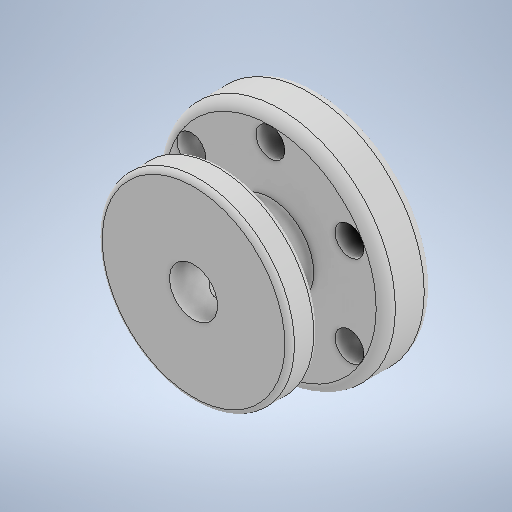
# Autodesk Inventor part: Steering Gear Plate 2
Saved by Autodesk Inventor 2025.2 (Build 292293000, 293)
## iProperties
Created: 2025-03-03
Part Number: Steering Gear Plate 2
Material: Generic
Document SubType Name: Modeling
Designer: eason
Density: 1 g/cm^3
Appearance: Default
Author: eason
Autodesk Inventor part; units mm, degrees
ref_plane "YZ Plane" through (0, 0, 0) normal (1, 0, 0) x (0, 1, 0)
sketch "Sketch1" plane through (0, 0, 0) normal (0, 0, 1) x (1, 0, 0)
  circle A0 centre (0, 0) radius 8
  circle A1 centre (0, 0) radius 11
  circle A2 centre (0, 9.5) radius 1.5
  line L0 (0, -15.4) -> (0, 15.4) projected
  circle A3 centre (-8.2272, 4.75) radius 1.5
  circle A4 centre (-8.2272, -4.75) radius 1.5
  circle A5 centre (0, -9.5) radius 1.5
  circle A6 centre (8.2272, -4.75) radius 1.5
  circle A7 centre (8.2272, 4.75) radius 1.5
  point P0 (-9.5263, 5.5)
  point P1 (-9.5263, -5.5)
  point P2 (9.5263, -5.5)
  point P3 (9.5263, 5.5)
  point P4 (0, 11)
  dimension "d0" = 16
  dimension "d1" = 22
  dimension "d4" = 360
  constraints: 8 centre point, 2 coincident, 2 tangent, 1 point on line, 13 other
  measures "d0" diameter of A0
  measures "d1" diameter of A1
extrude "Extrusion1" add sketch "Sketch1" along normal blind 5 contours A0 L0 | A0 A7 A1 A6 | A0 A2 A1 A7 | A6 A1 A5 A0 | L0 A0 | A0 A3 A1 A2 | A5 A1 A4 A0 | A5 L0 | L0 A5 | A0 A4 A1 A3
sketch "Sketch2" plane through (0, 0, 5) normal (0, 0, 1) x (1, 0, 0)
  circle A0 centre (0, 0) radius 10
  circle A1 centre (0, 0) radius 2.5
  dimension "d10" = 20
  dimension "d31" = 5
  constraints: 2 centre point, 2 coincident
  measures "d10" diameter of A0
  measures "d31" diameter of A1
extrude "Extrusion3" add sketch "Sketch2" along normal blind 8
extrude "Extrusion4" cut sketch "Sketch2" against normal through all contours A1
sketch "Sketch4" plane through (0, 0, 13) normal (0, 0, 1) x (1, 0, 0)
  line L0 (0, 0) -> (-3.4808, -9.3746) construction
  line L1 (0, -15.4) -> (0, 15.4) projected
  circle A0 centre (0, 0) radius 10 projected
  dimension "d16" = 20.37
  constraints: 2 end point, 2 other
  measures "d16" angle of L1 L0
ref_plane "Work Plane1" through (-3.4808, -9.3746, 13) normal (-0.3480812, -0.9374644, 0) x (0.9374644, -0.3480812, 0)
sketch "Sketch5" plane through (-3.4808, -9.3746, 13) normal (-0.3480812, -0.9374644, 0) x (0.9374644, -0.3480812, 0)
  circle A0 centre (0, -5) radius 1.5
  line L0 (10, 0) -> (-10, 0) projected
  line L1 (0, -15.6) -> (0, 2.6) projected
  line L2 (7.4257, -8) -> (10, -8) projected
  point P0 (0, -13)
  dimension "d17" = 3
  dimension "d33" = 3
  constraints: 1 centre point, 1 point on line
  measures "d17" diameter of A0
  measures "d33" distance from line of L2 A0.centre
extrude "Extrusion5" cut sketch "Sketch5" against normal up to surface
ref_plane "Work Plane2" through (0, 0, 9) normal (0, 0, 1) x (1, 0, 0)
sketch "Sketch6" plane through (0, 0, 9) normal (0, 0, 1) x (1, 0, 0)
  circle A0 centre (0, 0) radius 2.5 projected
  circle A1 centre (0, 0) radius 4.5
  circle A2 centre (0, 0) radius 10 projected
  dimension "d32" = 2
  constraints: 1 centre point, 1 coincident
  measures "d32" radial gap between concentric circles of A1 A0
extrude "Extrusion6" cut sketch "Sketch6" along normal blind 1 and the other way blind 4 contours A2
fillet "Fillet1" radius 0.5 6 edges at (-10, 0, 10) (-10, 0, 13) (-0.1708, -4.4968, 8.5251) (-1.5663, -4.2186, 9.5) (-2.1556, -3.9501, 6.6461) (-2.1024, -1.3528, 7.9953)
sketch "Sketch7" plane through (0, 0, 0) normal (0, 0, -1) x (-1, 0, 0)
  circle A0 centre (0, 0) radius 12
  arc A1 (9.5263, 5.5) -> (0, 11) centre (0, 0) ccw projected
  arc A2 (9.5263, -5.5) -> (9.5263, 5.5) centre (0, 0) ccw projected
  arc A3 (-9.5263, -5.5) -> (9.5263, -5.5) centre (0, 0) ccw projected
  arc A4 (-9.5263, 5.5) -> (-9.5263, -5.5) centre (0, 0) ccw projected
  arc A5 (0, 11) -> (-9.5263, 5.5) centre (0, 0) ccw projected
  arc A6 (9.5263, -5.5) -> (9.5263, 5.5) centre (0, 0) ccw projected
  circle A7 centre (8.2272, 4.75) radius 1.5 projected
  arc A8 (9.5263, 5.5) -> (0, 11) centre (0, 0) ccw projected
  circle A9 centre (0, 9.5) radius 1.5 projected
  arc A10 (0, 11) -> (-9.5263, 5.5) centre (0, 0) ccw projected
  circle A11 centre (-8.2272, 4.75) radius 1.5 projected
  arc A12 (-9.5263, 5.5) -> (-9.5263, -5.5) centre (0, 0) ccw projected
  circle A13 centre (-8.2272, -4.75) radius 1.5 projected
  arc A14 (-9.5263, -5.5) -> (9.5263, -5.5) centre (0, 0) ccw projected
  circle A15 centre (8.2272, -4.75) radius 1.5 projected
  dimension "d27" = 1
  constraints: 1 centre point, 1 coincident, 1 vertical alignment, 4 other
  measures "d27" radial gap between concentric circles of A1 A0
extrude "Extrusion7" add sketch "Sketch7" against normal up to surface (5 mm away) contours A0
fillet "Fillet2" radius 1 2 edges at (12, 0, 0) (12, 0, 5)
body "Solid1"
